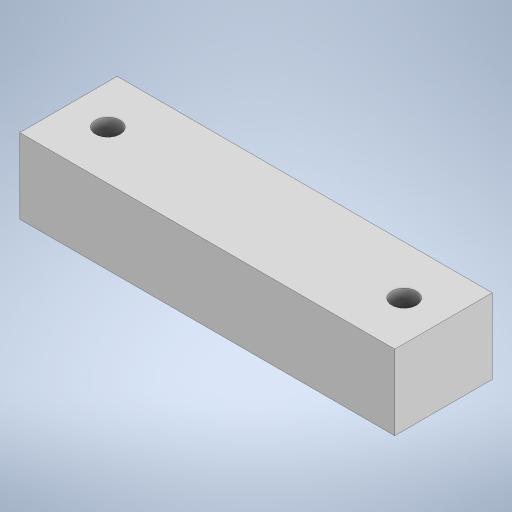
# Autodesk Inventor part: Conductor_RD16
Saved by Autodesk Inventor 2024 (Build 280153000, 153)
## iProperties
Created: 2024-11-17
Part Number: Conductor_RD16
Material: Типовые
Document SubType Name: Modeling
Designer: fm
Density: 1 g/cm^3
Appearance: По умолчанию
Author: fm
Autodesk Inventor part; units mm, degrees
ref_plane "YZ Plane" through (0, 0, 0) normal (1, 0, 0) x (0, 1, 0)
ref_plane "XZ Plane" through (0, 0, 0) normal (0, 1, 0) x (-1, 0, 0)
ref_plane "XY Plane" through (0, 0, 0) normal (0, 0, 1) x (1, 0, 0)
sketch "Эскиз1" plane through (0, 0, 0) normal (0, 1, 0) x (-1, 0, 0)
  line L0 (0, 0) -> (-50, 0)
  line L1 (-50, 0) -> (-50, 13)
  line L2 (-50, 13) -> (0, 13)
  line L3 (0, 13) -> (0, 0)
  line L4 (-50, 0) -> (0, 13) construction
  line L5 (-5.25, 6.5) -> (-44.75, 6.5) construction
  circle A0 centre (-5.25, 6.5) radius 1.65
  circle A1 centre (-44.75, 6.5) radius 1.65
  point P0 (-25, 6.5)
  point P1 (-25, 6.5)
  dimension "d0" = 50
  dimension "d1" = 13
  dimension "d2" = 39.5
  dimension "d3" = 3.3
  dimension "d4" = 3.3
  constraints: 12 end point, 4 coincident, 2 centre point, 2 horizontal, 2 midpoint, 2 parallel, 1 perpendicular
  measures "d0" distance of L1.end L2.end
  measures "d1" distance of L0.end L1.end
  measures "d2" distance of L5.start L5.end
  measures "d3" diameter of A0
  measures "d4" diameter of A1
extrude "Выдавливание1" add sketch "Эскиз1" along normal blind 10
